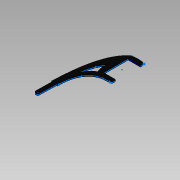
# Autodesk Inventor part: tibia
Saved by Autodesk Inventor 2015 SP1 (Build 190203100, 203)
## iProperties
Created: 2015-02-03
Part Number: tibia
Material: Generic
Document SubType Name: Modeling
Designer: Rafi Kurnia Putra
Density: 1 g/cm^3
Appearance: Smooth - Black
Author: Rafi Kurnia Putra
Autodesk Inventor part; units mm, degrees
ref_plane "YZ Plane" through (0, 0, 0) normal (1, 0, 0) x (0, 1, 0)
ref_plane "XZ Plane" through (0, 0, 0) normal (0, 1, 0) x (-1, 0, 0)
ref_plane "XY Plane" through (0, 0, 0) normal (0, 0, 1) x (1, 0, 0)
sketch "Sketch1" plane through (0, 0, 0) normal (0, 0, 1) x (1, 0, 0)
  line L0 (10.225, -20.79) -> (-10.225, -20.79)
  line L1 (-10.225, -20.79) -> (-10.225, 20.79)
  line L2 (-10.225, 20.79) -> (10.225, 20.79)
  line L3 (10.225, 20.79) -> (10.225, 26.79)
  circle A0 centre (5.065, 24.43) radius 1.1176
  circle A1 centre (-36.935, -103.5206) radius 1.65
  line L4 (10.225, -20.79) -> (10.225, -25.49)
  arc A2 (-40.1085, -104.2071) -> (-33.7294, -103.0042) centre (-36.935, -103.5206) ccw
  line L5 (-33.7294, -103.0042) -> (-33.01, -76.0171)
  line L6 (-40.1085, -104.2071) -> (-39.5798, -76.0171)
  line L7 (-33.01, -76.0171) -> (-31.71, -76.0171)
  line L8 (-39.5798, -76.0171) -> (-40.8798, -76.0171)
  arc A3 (8.225, -27.49) -> (10.225, -25.49) centre (8.225, -25.49) ccw
  line L9 (-31.71, -76.0171) -> (-31.71, -74.6543)
  line L10 (-40.8798, -76.0171) -> (-40.8798, -75.1175)
  spline S0 degree 2 poles (-40.8798, -75.1175) (-38.2166, 7.2621) (-10.775, 26.79) knots 0 0 0 1 1 1
  spline S1 degree 2 poles (-31.71, -74.6543) (-31.7475, -39.1438) (-10.225, -29.46) knots 0 0 0 1 1 1
  spline S2 degree 2 poles (-10.225, -29.46) (-3.1365, -27.3954) (8.225, -27.49) knots 0 0 0 1 1 1
  spline S3 degree 2 poles (-32.204, -45.7797) (-24.8502, -27.3026) (-16, -24.7698) knots 0 0 0 1 1 1
  spline S4 degree 2 poles (-16, -24.7698) (-20.1945, -14.9287) (-18.4094, -4.5078) knots 0 0 0 1 1 1
  spline S5 degree 2 poles (-32.204, -45.7797) (-29.4658, -17.3425) (-18.4094, -4.5078) knots 0 0 0 1 1 1
  circle A4 centre (-4.7394, 24.43) radius 1.1176
  circle A5 centre (5.065, -24.7698) radius 1.1176
  circle A6 centre (-4.7394, -24.7698) radius 1.1176
  spline S6 degree 2 poles (-10.775, 26.79) (-1.0049, 28.5095) (10.225, 26.79) knots 0 0 0 1 1 1
  line L11 (-39.5798, -76.0171) -> (-33.01, -76.0171)
  point P0 (0, 0)
  point P1 (-36.935, -65)
  point P2 (10.225, -27.49)
  point P3 (-36.935, -104.2071)
  point P4 (-27.9991, 3.0016)
  point P5 (-25, -42.9979)
  point P6 (-3.0564, -28.0484)
  point P7 (-22.7585, -29.2588)
  point P8 (-18.7033, -14.7527)
  point P9 (-26.4094, -18.5078)
  point P10 (-1, 27.6487)
  point P11 (-36.2948, -76.0171)
  dimension "d2" = 6
  dimension "d3" = 20.45
  dimension "d4" = 21
  dimension "d5" = 2.2352
  dimension "d6" = 5.16
  dimension "d7" = 3.64
  dimension "d8" = 42
  dimension "d9" = 3.3
  dimension "d11" = 42
  dimension "d12" = 8.67
  dimension "d17" = 1.3
  dimension "d18" = 1.3
  dimension "d19" = 6.7
  dimension "d20" = 2
  dimension "d21" = 2.2352
  dimension "d22" = 9.8044
  dimension "d23" = 2.2352
  dimension "d24" = 2.2352
  dimension "d25" = 9.8044
  dimension "d26" = 49.1998
  dimension "d34" = 131.9
  dimension "d35" = 3.285
  constraints: 24 end point, 7 centre point, 5 horizontal, 5 point on circle, 4 vertical, 2 horizontal alignment, 2 point on line, 1 parallel, 1 perpendicular, 1 tangent, 1 vertical alignment, 23 other
  measures "d2" distance of L2.end L3.end
  measures "d3" distance of L1.end L2.end
  measures "d4" distance of L3.end point (-10.775, 26.79)
  measures "d5" diameter of A0
  measures "d6" distance from line of L3 A0.centre
  measures "d7" distance from line of L2 A0.centre
  measures "d8" horizontal distance of point (-36.935, -65) A0.centre
  measures "d9" diameter of A1
  measures "d11" horizontal distance of A1.centre A0.centre
  measures "d12" distance from line of point (-10.225, -29.46) L0
  measures "d17" distance of L5.end L7.end
  measures "d18" distance of L6.end L8.end
  measures "d19" distance of L0.start point (10.225, -27.49)
  measures "d20" radius of A3
  measures "d21" diameter of A4
  measures "d22" distance of A4.centre A0.centre
  measures "d23" diameter of A5
  measures "d24" diameter of A6
  measures "d25" distance of A6.centre A5.centre
  measures "d26" distance of A5.centre A0.centre
  measures "d35" distance of point (-36.295, -76.017) L6.end
extrude "Extrusion1" add sketch "Sketch1" along normal mid plane 3.5 contours L4 A3 S2 S1 L9 L7 L11 L8 L10 S0 S6 L3 L2 L1 L0 | L5 A2 L6 L11 | A0 | A1 | S5 S4 S3 | A4 | A5 | A6
fillet "Fillet1" radius 9 2 edges at (-10.775, 26.79, 0.875) (-10.775, 26.79, -0.875)
fillet "Fillet2" radius 4 2 edges at (10.225, 26.79, 0.875) (10.225, 26.79, -0.875)
fillet "Fillet3" radius 0.25 4 edges at (10.225, -20.79, 0) (10.225, 20.79, 0) (-31.71, -76.0171, 0) (-40.8798, -76.0171, 0)
extrude "Extrusion2" cut sketch "Sketch1" along normal through all both and the other way through all contours A0 | A1 | S5 S4 S3 | A4 | A5 | A6
body "Solid1"
